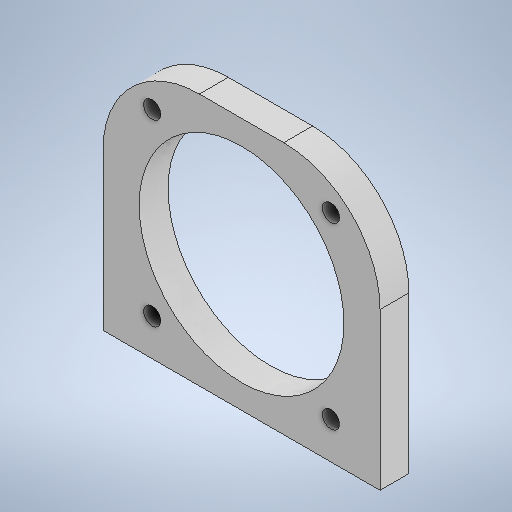
# Autodesk Inventor part: Gear_support_wheel
Saved by Autodesk Inventor 2025.2 (Build 292293000, 293)
## iProperties
Created: 2025-02-25
Part Number: Gear_support_wheel
Material: Generic
Document SubType Name: Modeling
Designer: Sergio Quintero
Density: 1 g/cm^3
Appearance: Default
Author: Sergio Quintero
Autodesk Inventor part; units mm, degrees
ref_plane "YZ Plane" through (0, 0, 0) normal (1, 0, 0) x (0, 1, 0)
ref_plane "XZ Plane" through (0, 0, 0) normal (0, 1, 0) x (-1, 0, 0)
ref_plane "XY Plane" through (0, 0, 0) normal (0, 0, 1) x (1, 0, 0)
sketch "Sketch1" plane through (0, 0, 0) normal (0, 0, 1) x (1, 0, 0)
  line L0 (57.5, -52.5) -> (-57.5, -52.5)
  line L1 (-57.5, -52.5) -> (-57.5, 52.5)
  line L2 (-57.5, 52.5) -> (57.5, 52.5)
  line L3 (57.5, 52.5) -> (57.5, -52.5)
  line L4 (57.5, -52.5) -> (-57.5, 52.5) construction
  line L5 (-57.5, -52.5) -> (57.5, 52.5) construction
  point P0 (0, 0)
  dimension "d0" = 115
  dimension "d1" = 105
  constraints: 12 end point, 2 midpoint, 2 parallel, 1 horizontal, 1 perpendicular
  measures "d0" distance of L1.end L2.end
  measures "d1" distance of L0.end L1.end
extrude "Extrusion1" add sketch "Sketch1" along normal blind 12
fillet "Fillet1" radius 40 2 edges at (-57.5, 52.5, 6) (57.5, 52.5, 6)
sketch "Sketch2" plane through (-57.5, -52.5, 0) normal (0, -1, 0) x (1, 0, 0)
  line L0 (0, 0) -> (0, 12) projected
  line L1 (115, 0) -> (115, 12) projected
  line L2 (0, 12) -> (115, 12) projected
  point P0 (57.5, 0)
  point P1 (10, 6)
  point P2 (105, 6)
  dimension "d5" = 10
  dimension "d6" = 10
  dimension "d7" = 6
  dimension "d8" = 6
  measures "d5" distance from line of L0 point (10, 6)
  measures "d6" distance from line of L1 point (105, 6)
  measures "d7" distance from line of L2 point (10, 6)
  measures "d8" distance from line of L2 point (105, 6)
hole "Hole1" at (-47.5, -52.5, 6) at (47.5, -52.5, 6) direction (0, 1, 0) diameter 7.134 depth 20.2 tip angle 118 thread size "M8x0.8" class "6H" standard "ISO Metric profile"
sketch "Sketch3" plane through (0, 0, 12) normal (0, 0, 1) x (1, 0, 0)
  circle A0 centre (0, 0) radius 42.5
  dimension "d16" = 85
  constraints: 1 centre point, 1 coincident
  measures "d16" diameter of A0
extrude "Extrusion2" cut sketch "Sketch3" against normal blind 12
sketch "Sketch4" plane through (0, 0, 12) normal (0, 0, 1) x (1, 0, 0)
  circle A0 centre (0, 0) radius 52.5 construction
  line L0 (0, 0) -> (-64.3477, 64.3477) construction
  line L1 (0, 0) -> (91.0013, 0) construction
  point P0 (-37.1231, 37.1231)
  dimension "d19" = 105
  dimension "d20" = 135
  constraints: 4 end point, 1 coincident, 1 equal length, 1 horizontal, 1 point on line, 3 other
  measures "d20" angle of L1 L0
hole "Hole2" at (-37.1231, 37.1231, 12) direction (0, 0, -1) diameter 7.134 depth 20.2 tip angle 118 thread size "M8x0.8" class "6H" standard "ISO Metric profile"
pattern_circular "Circular Pattern1" count 4 over 360 about axis through (0, 0, -10) along (0, 0, 1) of "Hole2"
body "Solid1"
